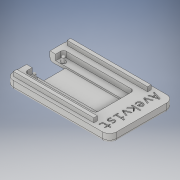
# Autodesk Inventor part: NodeMCU_Template
Saved by Autodesk Inventor 2019 (Build 230136000, 136)
## iProperties
Created: 2018-11-08
Part Number: NodeMCU_Template
Material: Generic
Document SubType Name: Modeling
Designer: hampu
Density: 1 g/cm^3
Appearance: Default
Author: hampu
Autodesk Inventor part; units mm, degrees
(part 1 of 2)
ref_plane "YZ Plane" through (0, 0, 0) normal (1, 0, 0) x (0, 1, 0)
ref_plane "XZ Plane" through (0, 0, 0) normal (0, 1, 0) x (-1, 0, 0)
ref_plane "XY Plane" through (0, 0, 0) normal (0, 0, 1) x (1, 0, 0)
sketch "Sketch1" plane through (0, 0, 0) normal (0, 1, 0) x (-1, 0, 0)
  line L0 (24.095, -12.775) -> (-24.095, -12.775)
  line L1 (-24.095, -12.775) -> (-24.095, 12.775)
  line L2 (-24.095, 12.775) -> (24.095, 12.775)
  line L3 (24.095, 12.775) -> (24.095, -12.775)
  line L4 (24.095, -12.775) -> (-24.095, 12.775) construction
  line L5 (-24.095, -12.775) -> (24.095, 12.775) construction
  line L6 (24.095, -12.775) -> (21.595, -12.775)
  line L7 (24.095, -12.775) -> (24.095, -10.275)
  line L8 (24.095, 12.775) -> (24.095, 10.275)
  line L9 (-24.095, -12.775) -> (-21.595, -12.775)
  line L10 (-24.095, 12.775) -> (-21.595, 12.775)
  line L11 (-24.095, 10.275) -> (-24.095, 12.775)
  circle A0 centre (21.595, -10.275) radius 1.7053
  circle A1 centre (-21.595, -10.275) radius 1.7053
  circle A2 centre (21.595, 10.275) radius 1.7053
  circle A3 centre (-21.595, 10.275) radius 1.7053
  point P0 (0, 0)
  dimension "d4" = 48.19
  dimension "d5" = 25.55
  dimension "d15" = 3.4106
  dimension "d18" = 43.19
  dimension "d21" = 20.55
  constraints: 24 end point, 4 centre point, 4 horizontal, 3 point on line, 2 midpoint, 2 parallel, 1 perpendicular, 1 vertical, 6 other
  measures "d4" distance of L0.start L0.end
  measures "d5" distance of L0.end L1.end
  measures "d15" diameter of A0
  measures "d18" distance of A0.centre A1.centre
  measures "d21" distance of A0.centre A2.centre
extrude "Extrusion2" add sketch "Sketch1" along normal blind 1.6
fillet "Fillet1" radius 2.5 4 edges at (-24.095, 0.8, 12.775) (-24.095, 0.8, -12.775) (24.095, 0.8, 12.775) (24.095, 0.8, -12.775)
sketch "Sketch3" plane through (0, 1.6, 0) normal (0, 1, 0) x (1, 0, 0)
  circle A0 centre (-21.595, 10.275) radius 1.7053 projected
  line L0 (21.595, 12.775) -> (-21.595, 12.775) projected
  line L1 (-19.1777, 12.775) -> (-18.624, 12.775) construction
  line L2 (-18.865, 12.2213) -> (-16.951, 12.2213)
  line L3 (-19.1777, 11.908) -> (-18.865, 12.2213)
  line L4 (-19.1777, 11.908) -> (-19.1777, 9.993)
  line L5 (-19.1777, 9.993) -> (-18.865, 9.6808)
  line L6 (-18.865, 9.6808) -> (-16.951, 9.6808)
  line L7 (-16.951, 9.6808) -> (-16.6393, 9.993)
  line L8 (-16.6393, 9.993) -> (-16.6393, 11.9102)
  line L9 (-18.226, 11.268) -> (-17.591, 11.268)
  line L10 (-17.591, 11.268) -> (-17.591, 10.633)
  line L11 (-17.591, 10.633) -> (-18.226, 10.633)
  line L12 (-18.226, 10.633) -> (-18.226, 11.268)
  line L13 (-16.951, 12.2213) -> (-16.6393, 11.9102)
  line L14 (-16.6377, 11.908) -> (-16.325, 12.2213)
  line L15 (-16.6377, 11.908) -> (-16.6377, 9.993)
  line L16 (-16.6377, 9.993) -> (-16.325, 9.6808)
  line L17 (-15.686, 10.633) -> (-15.686, 11.268)
  line L18 (-15.686, 11.268) -> (-15.051, 11.268)
  line L19 (-15.051, 11.268) -> (-15.051, 10.633)
  line L20 (-15.051, 10.633) -> (-15.686, 10.633)
  line L21 (-16.325, 9.6808) -> (-14.411, 9.6808)
  line L22 (-14.411, 9.6808) -> (-14.0993, 9.993)
  line L23 (-14.0993, 9.993) -> (-14.0993, 11.9102)
  line L24 (-14.411, 12.2213) -> (-14.0993, 11.9102)
  line L25 (-16.325, 12.2213) -> (-14.411, 12.2213)
  line L26 (-14.0977, 11.908) -> (-13.785, 12.2213)
  line L27 (-14.0977, 11.908) -> (-14.0977, 9.993)
  line L28 (-14.0977, 9.993) -> (-13.785, 9.6808)
  line L29 (-13.146, 10.633) -> (-13.146, 11.268)
  line L30 (-13.146, 11.268) -> (-12.511, 11.268)
  line L31 (-12.511, 11.268) -> (-12.511, 10.633)
  line L32 (-12.511, 10.633) -> (-13.146, 10.633)
  line L33 (-13.785, 9.6808) -> (-11.871, 9.6808)
  line L34 (-11.871, 9.6808) -> (-11.5593, 9.993)
  line L35 (-11.5593, 9.993) -> (-11.5593, 11.9102)
  line L36 (-11.871, 12.2213) -> (-11.5593, 11.9102)
  line L37 (-13.785, 12.2213) -> (-11.871, 12.2213)
  line L38 (-11.5577, 11.908) -> (-11.245, 12.2213)
  line L39 (-11.5577, 11.908) -> (-11.5577, 9.993)
  line L40 (-11.5577, 9.993) -> (-11.245, 9.6808)
  line L41 (-10.606, 10.633) -> (-10.606, 11.268)
  line L42 (-10.606, 11.268) -> (-9.971, 11.268)
  line L43 (-9.971, 11.268) -> (-9.971, 10.633)
  line L44 (-9.971, 10.633) -> (-10.606, 10.633)
  line L45 (-11.245, 9.6808) -> (-9.331, 9.6808)
  line L46 (-9.331, 9.6808) -> (-9.0193, 9.993)
  line L47 (-9.0193, 9.993) -> (-9.0193, 11.9102)
  line L48 (-9.331, 12.2213) -> (-9.0193, 11.9102)
  line L49 (-11.245, 12.2213) -> (-9.331, 12.2213)
  line L50 (-9.0177, 11.908) -> (-8.705, 12.2213)
  line L51 (-9.0177, 11.908) -> (-9.0177, 9.993)
  line L52 (-9.0177, 9.993) -> (-8.705, 9.6808)
  line L53 (-8.066, 10.633) -> (-8.066, 11.268)
  line L54 (-8.066, 11.268) -> (-7.431, 11.268)
  line L55 (-7.431, 11.268) -> (-7.431, 10.633)
  line L56 (-7.431, 10.633) -> (-8.066, 10.633)
  line L57 (-8.705, 9.6808) -> (-6.791, 9.6808)
  line L58 (-6.791, 9.6808) -> (-6.4793, 9.993)
  line L59 (-6.4793, 9.993) -> (-6.4793, 11.9102)
  line L60 (-6.791, 12.2213) -> (-6.4793, 11.9102)
  line L61 (-8.705, 12.2213) -> (-6.791, 12.2213)
  line L62 (-6.4777, 11.908) -> (-6.165, 12.2213)
  line L63 (-6.4777, 11.908) -> (-6.4777, 9.993)
  line L64 (-6.4777, 9.993) -> (-6.165, 9.6808)
  line L65 (-5.526, 10.633) -> (-5.526, 11.268)
  line L66 (-5.526, 11.268) -> (-4.891, 11.268)
  line L67 (-4.891, 11.268) -> (-4.891, 10.633)
  line L68 (-4.891, 10.633) -> (-5.526, 10.633)
  line L69 (-6.165, 9.6808) -> (-4.251, 9.6808)
  line L70 (-4.251, 9.6808) -> (-3.9393, 9.993)
  line L71 (-3.9393, 9.993) -> (-3.9393, 11.9102)
  line L72 (-4.251, 12.2213) -> (-3.9393, 11.9102)
  line L73 (-6.165, 12.2213) -> (-4.251, 12.2213)
  line L74 (-3.9377, 11.908) -> (-3.625, 12.2213)
  line L75 (-3.9377, 11.908) -> (-3.9377, 9.993)
  line L76 (-3.9377, 9.993) -> (-3.625, 9.6808)
  line L77 (-2.986, 10.633) -> (-2.986, 11.268)
  line L78 (-2.986, 11.268) -> (-2.351, 11.268)
  line L79 (-2.351, 11.268) -> (-2.351, 10.633)
  line L80 (-2.351, 10.633) -> (-2.986, 10.633)
  line L81 (-3.625, 9.6808) -> (-1.711, 9.6808)
  line L82 (-1.711, 9.6808) -> (-1.3993, 9.993)
  line L83 (-1.3993, 9.993) -> (-1.3993, 11.9102)
  line L84 (-1.711, 12.2213) -> (-1.3993, 11.9102)
  line L85 (-3.625, 12.2213) -> (-1.711, 12.2213)
  line L86 (-1.3977, 11.908) -> (-1.085, 12.2213)
  line L87 (-1.3977, 11.908) -> (-1.3977, 9.993)
  line L88 (-1.3977, 9.993) -> (-1.085, 9.6808)
  line L89 (-0.446, 10.633) -> (-0.446, 11.268)
  line L90 (-0.446, 11.268) -> (0.189, 11.268)
  line L91 (0.189, 11.268) -> (0.189, 10.633)
  line L92 (0.189, 10.633) -> (-0.446, 10.633)
  line L93 (-1.085, 9.6808) -> (0.829, 9.6808)
  line L94 (0.829, 9.6808) -> (1.1407, 9.993)
  line L95 (1.1407, 9.993) -> (1.1407, 11.9102)
  line L96 (0.829, 12.2213) -> (1.1407, 11.9102)
  line L97 (-1.085, 12.2213) -> (0.829, 12.2213)
  line L98 (1.1423, 11.908) -> (1.455, 12.2213)
  line L99 (1.1423, 11.908) -> (1.1423, 9.993)
  line L100 (1.1423, 9.993) -> (1.455, 9.6808)
  line L101 (2.094, 10.633) -> (2.094, 11.268)
  line L102 (2.094, 11.268) -> (2.729, 11.268)
  line L103 (2.729, 11.268) -> (2.729, 10.633)
  line L104 (2.729, 10.633) -> (2.094, 10.633)
  line L105 (1.455, 9.6808) -> (3.369, 9.6808)
  line L106 (3.369, 9.6808) -> (3.6807, 9.993)
  line L107 (3.6807, 9.993) -> (3.6807, 11.9102)
  line L108 (3.369, 12.2213) -> (3.6807, 11.9102)
  line L109 (1.455, 12.2213) -> (3.369, 12.2213)
  line L110 (3.6823, 11.908) -> (3.995, 12.2213)
  line L111 (3.6823, 11.908) -> (3.6823, 9.993)
  line L112 (3.6823, 9.993) -> (3.995, 9.6808)
  line L113 (4.634, 10.633) -> (4.634, 11.268)
  line L114 (4.634, 11.268) -> (5.269, 11.268)
  line L115 (5.269, 11.268) -> (5.269, 10.633)
  line L116 (5.269, 10.633) -> (4.634, 10.633)
  line L117 (3.995, 9.6808) -> (5.909, 9.6808)
  line L118 (5.909, 9.6808) -> (6.2207, 9.993)
  line L119 (6.2207, 9.993) -> (6.2207, 11.9102)
  line L120 (5.909, 12.2213) -> (6.2207, 11.9102)
  line L121 (3.995, 12.2213) -> (5.909, 12.2213)
  line L122 (6.2223, 11.908) -> (6.535, 12.2213)
  line L123 (6.2223, 11.908) -> (6.2223, 9.993)
  line L124 (6.2223, 9.993) -> (6.535, 9.6808)
  line L125 (7.174, 10.633) -> (7.174, 11.268)
  line L126 (7.174, 11.268) -> (7.809, 11.268)
  line L127 (7.809, 11.268) -> (7.809, 10.633)
  line L128 (7.809, 10.633) -> (7.174, 10.633)
  line L129 (6.535, 9.6808) -> (8.449, 9.6808)
  line L130 (8.449, 9.6808) -> (8.7607, 9.993)
  line L131 (8.7607, 9.993) -> (8.7607, 11.9102)
  line L132 (8.449, 12.2213) -> (8.7607, 11.9102)
  line L133 (6.535, 12.2213) -> (8.449, 12.2213)
  line L134 (8.7623, 11.908) -> (9.075, 12.2213)
  line L135 (8.7623, 11.908) -> (8.7623, 9.993)
  line L136 (8.7623, 9.993) -> (9.075, 9.6808)
  line L137 (9.714, 10.633) -> (9.714, 11.268)
  line L138 (9.714, 11.268) -> (10.349, 11.268)
  line L139 (10.349, 11.268) -> (10.349, 10.633)
  line L140 (10.349, 10.633) -> (9.714, 10.633)
  line L141 (9.075, 9.6808) -> (10.989, 9.6808)
  line L142 (10.989, 9.6808) -> (11.3007, 9.993)
  line L143 (11.3007, 9.993) -> (11.3007, 11.9102)
  line L144 (10.989, 12.2213) -> (11.3007, 11.9102)
  line L145 (9.075, 12.2213) -> (10.989, 12.2213)
  line L146 (11.3023, 11.908) -> (11.615, 12.2213)
  line L147 (11.3023, 11.908) -> (11.3023, 9.993)
  line L148 (11.3023, 9.993) -> (11.615, 9.6808)
  line L149 (12.254, 10.633) -> (12.254, 11.268)
  line L150 (12.254, 11.268) -> (12.889, 11.268)
  line L151 (12.889, 11.268) -> (12.889, 10.633)
  line L152 (12.889, 10.633) -> (12.254, 10.633)
  line L153 (11.615, 9.6808) -> (13.529, 9.6808)
  line L154 (13.529, 9.6808) -> (13.8407, 9.993)
  line L155 (13.8407, 9.993) -> (13.8407, 11.9102)
  line L156 (13.529, 12.2213) -> (13.8407, 11.9102)
  line L157 (11.615, 12.2213) -> (13.529, 12.2213)
  line L158 (13.8423, 11.908) -> (14.155, 12.2213)
  line L159 (13.8423, 11.908) -> (13.8423, 9.993)
  line L160 (13.8423, 9.993) -> (14.155, 9.6808)
  line L161 (14.794, 10.633) -> (14.794, 11.268)
  line L162 (14.794, 11.268) -> (15.429, 11.268)
  line L163 (15.429, 11.268) -> (15.429, 10.633)
  line L164 (15.429, 10.633) -> (14.794, 10.633)
  line L165 (14.155, 9.6808) -> (16.069, 9.6808)
  line L166 (16.069, 9.6808) -> (16.3807, 9.993)
  line L167 (16.3807, 9.993) -> (16.3807, 11.9102)
  line L168 (16.069, 12.2213) -> (16.3807, 11.9102)
  line L169 (14.155, 12.2213) -> (16.069, 12.2213)
  line L170 (16.3823, 11.908) -> (16.695, 12.2213)
  line L171 (16.3823, 11.908) -> (16.3823, 9.993)
  line L172 (16.3823, 9.993) -> (16.695, 9.6808)
  line L173 (17.334, 10.633) -> (17.334, 11.268)
  line L174 (17.334, 11.268) -> (17.969, 11.268)
  line L175 (17.969, 11.268) -> (17.969, 10.633)
  line L176 (17.969, 10.633) -> (17.334, 10.633)
  line L177 (16.695, 9.6808) -> (18.609, 9.6808)
  line L178 (18.609, 9.6808) -> (18.9207, 9.993)
  line L179 (18.9207, 9.993) -> (18.9207, 11.9102)
  line L180 (18.609, 12.2213) -> (18.9207, 11.9102)
  line L181 (16.695, 12.2213) -> (18.609, 12.2213)
  line L182 (-19.1777, -9.9934) -> (-18.865, -9.6801)
  line L183 (-19.1777, -9.9934) -> (-19.1777, -11.9084)
  line L184 (-19.1777, -11.9084) -> (-18.865, -12.2206)
  line L185 (-18.226, -11.2684) -> (-18.226, -10.6334)
  line L186 (-18.226, -10.6334) -> (-17.591, -10.6334)
  line L187 (-17.591, -10.6334) -> (-17.591, -11.2684)
  line L188 (-17.591, -11.2684) -> (-18.226, -11.2684)
  line L189 (-18.865, -12.2206) -> (-16.951, -12.2206)
  line L190 (-16.951, -12.2206) -> (-16.6393, -11.9084)
  line L191 (-16.6393, -11.9084) -> (-16.6393, -9.9912)
  line L192 (-16.951, -9.6801) -> (-16.6393, -9.9912)
  line L193 (-18.865, -9.6801) -> (-16.951, -9.6801)
  line L194 (-16.6377, -9.9934) -> (-16.325, -9.6801)
  line L195 (-16.6377, -9.9934) -> (-16.6377, -11.9084)
  line L196 (-16.6377, -11.9084) -> (-16.325, -12.2206)
  line L197 (-15.686, -11.2684) -> (-15.686, -10.6334)
  line L198 (-15.686, -10.6334) -> (-15.051, -10.6334)
  line L199 (-15.051, -10.6334) -> (-15.051, -11.2684)
  line L200 (-15.051, -11.2684) -> (-15.686, -11.2684)
  line L201 (-16.325, -12.2206) -> (-14.411, -12.2206)
  line L202 (-14.411, -12.2206) -> (-14.0993, -11.9084)
  line L203 (-14.0993, -11.9084) -> (-14.0993, -9.9912)
  line L204 (-14.411, -9.6801) -> (-14.0993, -9.9912)
  line L205 (-16.325, -9.6801) -> (-14.411, -9.6801)
  line L206 (-14.0977, -9.9934) -> (-13.785, -9.6801)
  line L207 (-14.0977, -9.9934) -> (-14.0977, -11.9084)
  line L208 (-14.0977, -11.9084) -> (-13.785, -12.2206)
  line L209 (-13.146, -11.2684) -> (-13.146, -10.6334)
  line L210 (-13.146, -10.6334) -> (-12.511, -10.6334)
  line L211 (-12.511, -10.6334) -> (-12.511, -11.2684)
  line L212 (-12.511, -11.2684) -> (-13.146, -11.2684)
  line L213 (-13.785, -12.2206) -> (-11.871, -12.2206)
  line L214 (-11.871, -12.2206) -> (-11.5593, -11.9084)
  line L215 (-11.5593, -11.9084) -> (-11.5593, -9.9912)
  line L216 (-11.871, -9.6801) -> (-11.5593, -9.9912)
  line L217 (-13.785, -9.6801) -> (-11.871, -9.6801)
  line L218 (-11.5577, -9.9934) -> (-11.245, -9.6801)
  line L219 (-11.5577, -9.9934) -> (-11.5577, -11.9084)
  line L220 (-11.5577, -11.9084) -> (-11.245, -12.2206)
  line L221 (-10.606, -11.2684) -> (-10.606, -10.6334)
  line L222 (-10.606, -10.6334) -> (-9.971, -10.6334)
  line L223 (-9.971, -10.6334) -> (-9.971, -11.2684)
  line L224 (-9.971, -11.2684) -> (-10.606, -11.2684)
  line L225 (-11.245, -12.2206) -> (-9.331, -12.2206)
  line L226 (-9.331, -12.2206) -> (-9.0193, -11.9084)
  line L227 (-9.0193, -11.9084) -> (-9.0193, -9.9912)
  line L228 (-9.331, -9.6801) -> (-9.0193, -9.9912)
  line L229 (-11.245, -9.6801) -> (-9.331, -9.6801)
  line L230 (-9.0177, -9.9934) -> (-8.705, -9.6801)
  line L231 (-9.0177, -9.9934) -> (-9.0177, -11.9084)
  line L232 (-9.0177, -11.9084) -> (-8.705, -12.2206)
  line L233 (-8.066, -11.2684) -> (-8.066, -10.6334)
  line L234 (-8.066, -10.6334) -> (-7.431, -10.6334)
  line L235 (-7.431, -10.6334) -> (-7.431, -11.2684)
  line L236 (-7.431, -11.2684) -> (-8.066, -11.2684)
  line L237 (-8.705, -12.2206) -> (-6.791, -12.2206)
  line L238 (-6.791, -12.2206) -> (-6.4793, -11.9084)
  line L239 (-6.4793, -11.9084) -> (-6.4793, -9.9912)
  line L240 (-6.791, -9.6801) -> (-6.4793, -9.9912)
  line L241 (-8.705, -9.6801) -> (-6.791, -9.6801)
  line L242 (-6.4777, -9.9934) -> (-6.165, -9.6801)
  line L243 (-6.4777, -9.9934) -> (-6.4777, -11.9084)
  line L244 (-6.4777, -11.9084) -> (-6.165, -12.2206)
  line L245 (-5.526, -11.2684) -> (-5.526, -10.6334)
  line L246 (-5.526, -10.6334) -> (-4.891, -10.6334)
  line L247 (-4.891, -10.6334) -> (-4.891, -11.2684)
  line L248 (-4.891, -11.2684) -> (-5.526, -11.2684)
  line L249 (-6.165, -12.2206) -> (-4.251, -12.2206)
  line L250 (-4.251, -12.2206) -> (-3.9393, -11.9084)
  line L251 (-3.9393, -11.9084) -> (-3.9393, -9.9912)
  line L252 (-4.251, -9.6801) -> (-3.9393, -9.9912)
  line L253 (-6.165, -9.6801) -> (-4.251, -9.6801)
  line L254 (-3.9377, -9.9934) -> (-3.625, -9.6801)
  line L255 (-3.9377, -9.9934) -> (-3.9377, -11.9084)
  line L256 (-3.9377, -11.9084) -> (-3.625, -12.2206)
  line L257 (-2.986, -11.2684) -> (-2.986, -10.6334)
  line L258 (-2.986, -10.6334) -> (-2.351, -10.6334)
  line L259 (-2.351, -10.6334) -> (-2.351, -11.2684)
  line L260 (-2.351, -11.2684) -> (-2.986, -11.2684)
  line L261 (-3.625, -12.2206) -> (-1.711, -12.2206)
  line L262 (-1.711, -12.2206) -> (-1.3993, -11.9084)
  line L263 (-1.3993, -11.9084) -> (-1.3993, -9.9912)
  line L264 (-1.711, -9.6801) -> (-1.3993, -9.9912)
  line L265 (-3.625, -9.6801) -> (-1.711, -9.6801)
  line L266 (-1.3977, -9.9934) -> (-1.085, -9.6801)
  line L267 (-1.3977, -9.9934) -> (-1.3977, -11.9084)
  line L268 (-1.3977, -11.9084) -> (-1.085, -12.2206)
  line L269 (-0.446, -11.2684) -> (-0.446, -10.6334)
  line L270 (-0.446, -10.6334) -> (0.189, -10.6334)
  line L271 (0.189, -10.6334) -> (0.189, -11.2684)
  line L272 (0.189, -11.2684) -> (-0.446, -11.2684)
  line L273 (-1.085, -12.2206) -> (0.829, -12.2206)
  line L274 (0.829, -12.2206) -> (1.1407, -11.9084)
  line L275 (1.1407, -11.9084) -> (1.1407, -9.9912)
  line L276 (0.829, -9.6801) -> (1.1407, -9.9912)
  line L277 (-1.085, -9.6801) -> (0.829, -9.6801)
  line L278 (1.1423, -9.9934) -> (1.455, -9.6801)
  line L279 (1.1423, -9.9934) -> (1.1423, -11.9084)
  line L280 (1.1423, -11.9084) -> (1.455, -12.2206)
  line L281 (2.094, -11.2684) -> (2.094, -10.6334)
  line L282 (2.094, -10.6334) -> (2.729, -10.6334)
  line L283 (2.729, -10.6334) -> (2.729, -11.2684)
  line L284 (2.729, -11.2684) -> (2.094, -11.2684)
  line L285 (1.455, -12.2206) -> (3.369, -12.2206)
  line L286 (3.369, -12.2206) -> (3.6807, -11.9084)
  line L287 (3.6807, -11.9084) -> (3.6807, -9.9912)
  line L288 (3.369, -9.6801) -> (3.6807, -9.9912)
  line L289 (1.455, -9.6801) -> (3.369, -9.6801)
  line L290 (3.6823, -9.9934) -> (3.995, -9.6801)
  line L291 (3.6823, -9.9934) -> (3.6823, -11.9084)
  line L292 (3.6823, -11.9084) -> (3.995, -12.2206)
  line L293 (4.634, -11.2684) -> (4.634, -10.6334)
  line L294 (4.634, -10.6334) -> (5.269, -10.6334)
  line L295 (5.269, -10.6334) -> (5.269, -11.2684)
  line L296 (5.269, -11.2684) -> (4.634, -11.2684)
  line L297 (3.995, -12.2206) -> (5.909, -12.2206)
  line L298 (5.909, -12.2206) -> (6.2207, -11.9084)
  line L299 (6.2207, -11.9084) -> (6.2207, -9.9912)
  line L300 (5.909, -9.6801) -> (6.2207, -9.9912)
  line L301 (3.995, -9.6801) -> (5.909, -9.6801)
  line L302 (6.2223, -9.9934) -> (6.535, -9.6801)
  line L303 (6.2223, -9.9934) -> (6.2223, -11.9084)
  line L304 (6.2223, -11.9084) -> (6.535, -12.2206)
  line L305 (7.174, -11.2684) -> (7.174, -10.6334)
  line L306 (7.174, -10.6334) -> (7.809, -10.6334)
  line L307 (7.809, -10.6334) -> (7.809, -11.2684)
  line L308 (7.809, -11.2684) -> (7.174, -11.2684)
  line L309 (6.535, -12.2206) -> (8.449, -12.2206)
  line L310 (8.449, -12.2206) -> (8.7607, -11.9084)
  line L311 (8.7607, -11.9084) -> (8.7607, -9.9912)
  line L312 (8.449, -9.6801) -> (8.7607, -9.9912)
  line L313 (6.535, -9.6801) -> (8.449, -9.6801)
  line L314 (8.7623, -9.9934) -> (9.075, -9.6801)
  line L315 (8.7623, -9.9934) -> (8.7623, -11.9084)
  line L316 (8.7623, -11.9084) -> (9.075, -12.2206)
  line L317 (9.714, -11.2684) -> (9.714, -10.6334)
  line L318 (9.714, -10.6334) -> (10.349, -10.6334)
  line L319 (10.349, -10.6334) -> (10.349, -11.2684)
  line L320 (10.349, -11.2684) -> (9.714, -11.2684)
  line L321 (9.075, -12.2206) -> (10.989, -12.2206)
  line L322 (10.989, -12.2206) -> (11.3007, -11.9084)
  line L323 (11.3007, -11.9084) -> (11.3007, -9.9912)
  line L324 (10.989, -9.6801) -> (11.3007, -9.9912)
  line L325 (9.075, -9.6801) -> (10.989, -9.6801)
  line L326 (11.3023, -9.9934) -> (11.615, -9.6801)
  line L327 (11.3023, -9.9934) -> (11.3023, -11.9084)
  line L328 (11.3023, -11.9084) -> (11.615, -12.2206)
  line L329 (12.254, -11.2684) -> (12.254, -10.6334)
  line L330 (12.254, -10.6334) -> (12.889, -10.6334)
  line L331 (12.889, -10.6334) -> (12.889, -11.2684)
  line L332 (12.889, -11.2684) -> (12.254, -11.2684)
  line L333 (11.615, -12.2206) -> (13.529, -12.2206)
  line L334 (13.529, -12.2206) -> (13.8407, -11.9084)
  line L335 (13.8407, -11.9084) -> (13.8407, -9.9912)
  line L336 (13.529, -9.6801) -> (13.8407, -9.9912)
  line L337 (11.615, -9.6801) -> (13.529, -9.6801)
  line L338 (13.8423, -9.9934) -> (14.155, -9.6801)
  line L339 (13.8423, -9.9934) -> (13.8423, -11.9084)
  line L340 (13.8423, -11.9084) -> (14.155, -12.2206)
  line L341 (14.794, -11.2684) -> (14.794, -10.6334)
  line L342 (14.794, -10.6334) -> (15.429, -10.6334)
  line L343 (15.429, -10.6334) -> (15.429, -11.2684)
  line L344 (15.429, -11.2684) -> (14.794, -11.2684)
  line L345 (14.155, -12.2206) -> (16.069, -12.2206)
  line L346 (16.069, -12.2206) -> (16.3807, -11.9084)
  line L347 (16.3807, -11.9084) -> (16.3807, -9.9912)
  line L348 (16.069, -9.6801) -> (16.3807, -9.9912)
  line L349 (14.155, -9.6801) -> (16.069, -9.6801)
  line L350 (16.3823, -9.9934) -> (16.695, -9.6801)
  line L351 (16.3823, -9.9934) -> (16.3823, -11.9084)
  line L352 (16.3823, -11.9084) -> (16.695, -12.2206)
  line L353 (17.334, -11.2684) -> (17.334, -10.6334)
  line L354 (17.334, -10.6334) -> (17.969, -10.6334)
  line L355 (17.969, -10.6334) -> (17.969, -11.2684)
  line L356 (17.969, -11.2684) -> (17.334, -11.2684)
  line L357 (16.695, -12.2206) -> (18.609, -12.2206)
  line L358 (18.609, -12.2206) -> (18.9207, -11.9084)
  line L359 (18.9207, -11.9084) -> (18.9207, -9.9912)
  line L360 (18.609, -9.6801) -> (18.9207, -9.9912)
  line L361 (16.695, -9.6801) -> (18.609, -9.6801)
  point P0 (0, 0)
  dimension "d71" = 1.914
  dimension "d72" = 1.915
  dimension "d73" = 0.635
  dimension "d74" = 0.635
  dimension "d77" = 2.54
  dimension "d80" = 21.9014
  constraints: 722 end point, 4 horizontal, 4 perpendicular, 3 parallel, 2 collinear, 2 vertical, 1 point on line, 694 other
  measures "d71" distance of L2.start L2.end
  measures "d72" distance of L3.start L4.end
  measures "d73" distance of L10.end L11.end
  measures "d74" distance of L9.end L10.end
  measures "d77" distance of L3.start L14.start
  measures "d80" distance of L3.start L182.start
extrude "Extrusion3" add sketch "Sketch3" along normal blind 1.905 contours L2 L13 L8 L7 L6 L5 L4 L3 | L14 L25 L24 L23 L22 L21 L16 L8 | L26 L37 L36 L35 L34 L33 L28 L23 | L38 L49 L48 L47 L46 L45 L40 L35 | L50 L61 L60 L59 L58 L57 L52 L47 | L62 L73 L72 L71 L70 L69 L64 L59 | L74 L85 L84 L83 L82 L81 L76 L71 | L86 L97 L96 L95 L94 L93 L88 L83 | L98 L109 L108 L107 L106 L105 L100 L95 | L110 L121 L120 L119 L118 L117 L112 L107 | L122 L133 L132 L131 L130 L129 L124 L119 | L134 L145 L144 L143 L142 L141 L136 L131 | L146 L157 L156 L155 L154 L153 L148 L143 | L158 L169 L168 L167 L166 L165 L160 L155 | L170 L181 L180 L179 L178 L177 L172 L167 | L182 L193 L192 L191 L190 L189 L184 L183 | L194 L205 L204 L203 L202 L201 L196 L191 | L206 L217 L216 L215 L214 L213 L208 L203 | L218 L229 L228 L227 L226 L225 L220 L215 | L230 L241 L240 L239 L238 L237 L232 L227 | L242 L253 L252 L251 L250 L249 L244 L239 | L254 L265 L264 L263 L262 L261 L256 L251 | L266 L277 L276 L275 L274 L273 L268 L263 | L278 L289 L288 L287 L286 L285 L280 L275 | L290 L301 L300 L299 L298 L297 L292 L287 | L302 L313 L312 L311 L310 L309 L304 L299 | L314 L325 L324 L323 L322 L321 L316 L311 | L326 L337 L336 L335 L334 L333 L328 L323 | L338 L349 L348 L347 L346 L345 L340 L335 | L350 L361 L360 L359 L358 L357 L352 L347
sketch "Sketch4" plane through (0, 3.505, 0) normal (0, 1, 0) x (1, 0, 0)
  line L0 (-18.226, 10.633) -> (-18.226, 11.268) projected
  line L1 (-17.591, 10.633) -> (-17.591, 11.268) projected
  line L2 (-18.226, 11.268) -> (-17.591, 11.268)
  line L3 (-17.591, 11.268) -> (-17.591, 10.633)
  line L4 (-17.591, 10.633) -> (-18.226, 10.633)
  line L5 (-18.226, 10.633) -> (-18.226, 11.268)
  line L6 (-15.051, 11.268) -> (-15.051, 10.633)
  line L7 (-15.686, 11.268) -> (-15.051, 11.268)
  line L8 (-15.686, 10.633) -> (-15.686, 11.268)
  line L9 (-15.051, 10.633) -> (-15.686, 10.633)
  line L10 (-12.511, 11.268) -> (-12.511, 10.633)
  line L11 (-13.146, 11.268) -> (-12.511, 11.268)
  line L12 (-13.146, 10.633) -> (-13.146, 11.268)
  line L13 (-12.511, 10.633) -> (-13.146, 10.633)
  line L14 (-9.971, 11.268) -> (-9.971, 10.633)
  line L15 (-10.606, 11.268) -> (-9.971, 11.268)
  line L16 (-10.606, 10.633) -> (-10.606, 11.268)
  line L17 (-9.971, 10.633) -> (-10.606, 10.633)
  line L18 (-7.431, 11.268) -> (-7.431, 10.633)
  line L19 (-8.066, 11.268) -> (-7.431, 11.268)
  line L20 (-8.066, 10.633) -> (-8.066, 11.268)
  line L21 (-7.431, 10.633) -> (-8.066, 10.633)
  line L22 (-4.891, 11.268) -> (-4.891, 10.633)
  line L23 (-5.526, 11.268) -> (-4.891, 11.268)
  line L24 (-5.526, 10.633) -> (-5.526, 11.268)
  line L25 (-4.891, 10.633) -> (-5.526, 10.633)
  line L26 (-2.351, 11.268) -> (-2.351, 10.633)
  line L27 (-2.986, 11.268) -> (-2.351, 11.268)
  line L28 (-2.986, 10.633) -> (-2.986, 11.268)
  line L29 (-2.351, 10.633) -> (-2.986, 10.633)
  line L30 (0.189, 11.268) -> (0.189, 10.633)
  line L31 (-0.446, 11.268) -> (0.189, 11.268)
  line L32 (-0.446, 10.633) -> (-0.446, 11.268)
  line L33 (0.189, 10.633) -> (-0.446, 10.633)
  line L34 (2.729, 11.268) -> (2.729, 10.633)
  line L35 (2.094, 11.268) -> (2.729, 11.268)
  line L36 (2.094, 10.633) -> (2.094, 11.268)
  line L37 (2.729, 10.633) -> (2.094, 10.633)
  line L38 (5.269, 11.268) -> (5.269, 10.633)
  line L39 (4.634, 11.268) -> (5.269, 11.268)
  line L40 (4.634, 10.633) -> (4.634, 11.268)
  line L41 (5.269, 10.633) -> (4.634, 10.633)
  line L42 (7.809, 11.268) -> (7.809, 10.633)
  line L43 (7.174, 11.268) -> (7.809, 11.268)
  line L44 (7.174, 10.633) -> (7.174, 11.268)
  line L45 (7.809, 10.633) -> (7.174, 10.633)
  line L46 (10.349, 11.268) -> (10.349, 10.633)
  line L47 (9.714, 11.268) -> (10.349, 11.268)
  line L48 (9.714, 10.633) -> (9.714, 11.268)
  line L49 (10.349, 10.633) -> (9.714, 10.633)
  line L50 (12.889, 11.268) -> (12.889, 10.633)
  line L51 (12.254, 11.268) -> (12.889, 11.268)
  line L52 (12.254, 10.633) -> (12.254, 11.268)
  line L53 (12.889, 10.633) -> (12.254, 10.633)
  line L54 (15.429, 11.268) -> (15.429, 10.633)
  line L55 (14.794, 11.268) -> (15.429, 11.268)
  line L56 (14.794, 10.633) -> (14.794, 11.268)
  line L57 (15.429, 10.633) -> (14.794, 10.633)
  line L58 (17.969, 11.268) -> (17.969, 10.633)
  line L59 (17.334, 11.268) -> (17.969, 11.268)
  line L60 (17.334, 10.633) -> (17.334, 11.268)
  line L61 (17.969, 10.633) -> (17.334, 10.633)
  line L62 (-17.591, -10.6334) -> (-17.591, -11.2684)
  line L63 (-18.226, -10.6334) -> (-17.591, -10.6334)
  line L64 (-18.226, -11.2684) -> (-18.226, -10.6334)
  line L65 (-17.591, -11.2684) -> (-18.226, -11.2684)
  line L66 (-15.051, -10.6334) -> (-15.051, -11.2684)
  line L67 (-15.686, -10.6334) -> (-15.051, -10.6334)
  line L68 (-15.686, -11.2684) -> (-15.686, -10.6334)
  line L69 (-15.051, -11.2684) -> (-15.686, -11.2684)
  line L70 (-12.511, -10.6334) -> (-12.511, -11.2684)
  line L71 (-13.146, -10.6334) -> (-12.511, -10.6334)
  line L72 (-13.146, -11.2684) -> (-13.146, -10.6334)
  line L73 (-12.511, -11.2684) -> (-13.146, -11.2684)
  line L74 (-9.971, -10.6334) -> (-9.971, -11.2684)
  line L75 (-10.606, -10.6334) -> (-9.971, -10.6334)
  line L76 (-10.606, -11.2684) -> (-10.606, -10.6334)
  line L77 (-9.971, -11.2684) -> (-10.606, -11.2684)
  line L78 (-7.431, -10.6334) -> (-7.431, -11.2684)
  line L79 (-8.066, -10.6334) -> (-7.431, -10.6334)
  line L80 (-8.066, -11.2684) -> (-8.066, -10.6334)
  line L81 (-7.431, -11.2684) -> (-8.066, -11.2684)
  line L82 (-4.891, -10.6334) -> (-4.891, -11.2684)
  line L83 (-5.526, -10.6334) -> (-4.891, -10.6334)
  line L84 (-5.526, -11.2684) -> (-5.526, -10.6334)
  line L85 (-4.891, -11.2684) -> (-5.526, -11.2684)
  line L86 (-2.351, -10.6334) -> (-2.351, -11.2684)
  line L87 (-2.986, -10.6334) -> (-2.351, -10.6334)
  line L88 (-2.986, -11.2684) -> (-2.986, -10.6334)
  line L89 (-2.351, -11.2684) -> (-2.986, -11.2684)
  line L90 (0.189, -10.6334) -> (0.189, -11.2684)
  line L91 (-0.446, -10.6334) -> (0.189, -10.6334)
  line L92 (-0.446, -11.2684) -> (-0.446, -10.6334)
  line L93 (0.189, -11.2684) -> (-0.446, -11.2684)
  line L94 (2.729, -10.6334) -> (2.729, -11.2684)
  line L95 (2.094, -10.6334) -> (2.729, -10.6334)
  line L96 (2.094, -11.2684) -> (2.094, -10.6334)
  line L97 (2.729, -11.2684) -> (2.094, -11.2684)
  line L98 (5.269, -10.6334) -> (5.269, -11.2684)
  line L99 (4.634, -10.6334) -> (5.269, -10.6334)
  line L100 (4.634, -11.2684) -> (4.634, -10.6334)
  line L101 (5.269, -11.2684) -> (4.634, -11.2684)
  line L102 (7.809, -10.6334) -> (7.809, -11.2684)
  line L103 (7.174, -10.6334) -> (7.809, -10.6334)
  line L104 (7.174, -11.2684) -> (7.174, -10.6334)
  line L105 (7.809, -11.2684) -> (7.174, -11.2684)
  line L106 (10.349, -10.6334) -> (10.349, -11.2684)
  line L107 (9.714, -10.6334) -> (10.349, -10.6334)
  line L108 (9.714, -11.2684) -> (9.714, -10.6334)
  line L109 (10.349, -11.2684) -> (9.714, -11.2684)
  line L110 (12.889, -10.6334) -> (12.889, -11.2684)
  line L111 (12.254, -10.6334) -> (12.889, -10.6334)
  line L112 (12.254, -11.2684) -> (12.254, -10.6334)
  line L113 (12.889, -11.2684) -> (12.254, -11.2684)
  line L114 (15.429, -10.6334) -> (15.429, -11.2684)
  line L115 (14.794, -10.6334) -> (15.429, -10.6334)
  line L116 (14.794, -11.2684) -> (14.794, -10.6334)
  line L117 (15.429, -11.2684) -> (14.794, -11.2684)
  line L118 (17.969, -10.6334) -> (17.969, -11.2684)
  line L119 (17.334, -10.6334) -> (17.969, -10.6334)
  line L120 (17.334, -11.2684) -> (17.334, -10.6334)
  line L121 (17.969, -11.2684) -> (17.334, -11.2684)
  point P0 (0, 0)
  dimension "d89" = 2.54
  dimension "d92" = 21.9014
  constraints: 240 end point, 2 horizontal, 2 parallel, 1 collinear, 1 perpendicular, 1 vertical, 231 other
  measures "d89" distance of L2.end L6.start
  measures "d92" distance of L2.end L62.start
extrude "Extrusion5" add sketch "Sketch4" along normal blind 6.1913
chamfer "Chamfer1" distance 0.2 angle 45 120 edges at (-17.591, 9.6963, 10.9509) (-18.226, 9.6963, 10.9509) (-17.9085, 9.6963, 11.2684) (-17.9085, 9.6963, 10.6334) (-15.686, 9.6963, 10.9509) (-15.3685, 9.6963, 11.2684) (-15.051, 9.6963, 10.9509) (-15.3685, 9.6963, 10.6334) (-13.146, 9.6963, 10.9509) (-12.8285, 9.6963, 10.6334) (-12.511, 9.6963, 10.9509) (-12.8285, 9.6963, 11.2684) (-10.606, 9.6963, 10.9509) (-10.2885, 9.6963, 11.2684) (-9.971, 9.6963, 10.9509) (-10.2885, 9.6963, 10.6334) (-7.431, 9.6963, 10.9509) (-7.7485, 9.6963, 11.2684) (-8.066, 9.6963, 10.9509) (-7.7485, 9.6963, 10.6334) (-5.526, 9.6963, 10.9509) (-5.2085, 9.6963, 10.6334) (-4.891, 9.6963, 10.9509) (-5.2085, 9.6963, 11.2684) (-2.986, 9.6963, 10.9509) (-2.6685, 9.6963, 10.6334) (-2.6685, 9.6963, 11.2684) (-2.351, 9.6963, 10.9509) (-0.446, 9.6963, 10.9509) (-0.1285, 9.6963, 10.6334) (0.189, 9.6963, 10.9509) (-0.1285, 9.6963, 11.2684) (2.4115, 9.6963, 11.2684) (2.094, 9.6963, 10.9509) (2.4115, 9.6963, 10.6334) (2.729, 9.6963, 10.9509) (5.269, 9.6963, 10.9509) (4.9515, 9.6963, 11.2684) (4.634, 9.6963, 10.9509) (4.9515, 9.6963, 10.6334) (7.809, 9.6963, 10.9509) (7.4915, 9.6963, 11.2684) (7.174, 9.6963, 10.9509) (7.4915, 9.6963, 10.6334) (9.714, 9.6963, 10.9509) (10.0315, 9.6963, 10.6334) (10.349, 9.6963, 10.9509) (10.0315, 9.6963, 11.2684) (12.5715, 9.6963, 11.2684) (12.889, 9.6963, 10.9509) (12.5715, 9.6963, 10.6334) (12.254, 9.6963, 10.9509) (14.794, 9.6963, 10.9509) (15.1115, 9.6963, 10.6334) (15.429, 9.6963, 10.9509) (15.1115, 9.6963, 11.2684) (17.6515, 9.6963, 11.2684) (17.969, 9.6963, 10.9509) (17.6515, 9.6963, 10.6334) (17.334, 9.6963, 10.9509) (-18.226, 9.6963, -10.9505) (-17.9085, 9.6963, -11.268) (-17.591, 9.6963, -10.9505) (-17.9085, 9.6963, -10.633) (-15.686, 9.6963, -10.9505) (-15.3685, 9.6963, -11.268) (-15.051, 9.6963, -10.9505) (-15.3685, 9.6963, -10.633) (-13.146, 9.6963, -10.9505) (-12.8285, 9.6963, -11.268) (-12.511, 9.6963, -10.9505) (-12.8285, 9.6963, -10.633) (-10.606, 9.6963, -10.9505) (-10.2885, 9.6963, -10.633) (-9.971, 9.6963, -10.9505) (-10.2885, 9.6963, -11.268) (-8.066, 9.6963, -10.9505) (-7.7485, 9.6963, -11.268) (-7.431, 9.6963, -10.9505) (-7.7485, 9.6963, -10.633) (-5.526, 9.6963, -10.9505) (-5.2085, 9.6963, -10.633) (-4.891, 9.6963, -10.9505) (-5.2085, 9.6963, -11.268) (-2.986, 9.6963, -10.9505) (-2.6685, 9.6963, -10.633) (-2.6685, 9.6963, -11.268) (-2.351, 9.6963, -10.9505) (-0.446, 9.6963, -10.9505) (-0.1285, 9.6963, -11.268) (0.189, 9.6963, -10.9505) (-0.1285, 9.6963, -10.633) (2.094, 9.6963, -10.9505) (2.4115, 9.6963, -11.268) (2.729, 9.6963, -10.9505) (2.4115, 9.6963, -10.633) (4.634, 9.6963, -10.9505) (4.9515, 9.6963, -11.268) (4.9515, 9.6963, -10.633) (5.269, 9.6963, -10.9505) (7.174, 9.6963, -10.9505) (7.4915, 9.6963, -10.633) (7.809, 9.6963, -10.9505) (7.4915, 9.6963, -11.268) (10.0315, 9.6963, -11.268) (9.714, 9.6963, -10.9505) (10.0315, 9.6963, -10.633) (10.349, 9.6963, -10.9505) (12.254, 9.6963, -10.9505) (12.5715, 9.6963, -11.268) (12.5715, 9.6963, -10.633) (12.889, 9.6963, -10.9505) (15.1115, 9.6963, -11.268) (15.429, 9.6963, -10.9505) (15.1115, 9.6963, -10.633) (14.794, 9.6963, -10.9505) (17.334, 9.6963, -10.9505) (17.6515, 9.6963, -10.633) (17.969, 9.6963, -10.9505) (17.6515, 9.6963, -11.268)
sketch "Sketch5" plane through (0, 0, 0) normal (0, -1, 0) x (1, 0, 0)
  line L0 (17.5, -10) -> (-17.5, -10)
  line L1 (-17.5, -10) -> (-17.5, 10)
  line L2 (-17.5, 10) -> (17.5, 10)
  line L3 (17.5, 10) -> (17.5, -10)
  line L4 (17.5, -10) -> (-17.5, 10) construction
  line L5 (-17.5, -10) -> (17.5, 10) construction
  point P0 (0, 0)
  dimension "d100" = 35
  dimension "d101" = 20
  constraints: 12 end point, 2 midpoint, 2 parallel, 1 horizontal, 1 perpendicular
  measures "d100" distance of L1.end L2.end
  measures "d101" distance of L0.end L1.end
extrude "Extrusion6" add sketch "Sketch5" along normal blind 2.5
sketch "Sketch6" plane through (0, -2.5, 0) normal (0, -1, 0) x (1, 0, 0)
  line L0 (24.095, -12.775) -> (-24.095, -12.775)
  line L1 (-24.095, -12.775) -> (-24.095, 12.775)
  line L2 (-24.095, 12.775) -> (24.095, 12.775)
  line L3 (24.095, 12.775) -> (24.095, -12.775)
  line L4 (24.095, -12.775) -> (-24.095, 12.775) construction
  line L5 (-24.095, -12.775) -> (24.095, 12.775) construction
  point P0 (0, 0)
  constraints: 12 end point, 2 midpoint, 2 parallel, 1 horizontal, 1 perpendicular
extrude "Extrusion7" add sketch "Sketch6" against normal blind 3
sketch "Sketch7" plane through (-21.595, 0.5, -10.275) normal (0, 1, 0) x (1, 0, 0)
  circle A0 centre (0, 0) radius 1.7053
  circle A1 centre (0, -20.55) radius 1.7053 projected
  circle A2 centre (0, -20.55) radius 1.7053
  point P0 (21.595, -10.275)
  constraints: 2 centre point, 1 coincident
extrude "Extrusion8" cut sketch "Sketch7" against normal blind 3
sketch "Sketch8" plane through (-24.095, 1.6, -10.275) normal (-1, 0, 0) x (0, 0, 1)
  line L0 (-2.5, -4.1) -> (23.05, -4.1) projected
  line L1 (2, -2) -> (18.55, -2)
  line L2 (18.55, -2) -> (18.55, -4.1)
  line L3 (18.55, -4.1) -> (2, -4.1)
  line L4 (2, -4.1) -> (2, -2)
  point P0 (10.275, -1.6)
  dimension "d108" = 16.55
  constraints: 8 end point, 2 parallel, 1 horizontal, 1 perpendicular, 1 point on line
  measures "d108" distance of L2.end L3.end
extrude "Extrusion9" cut sketch "Sketch8" against normal blind 8
sketch "Sketch9" plane through (-24.095, 1.6, -10.275) normal (-1, 0, 0) x (0, 0, 1)
  line L0 (-2.5, -4.1) -> (2, -4.1) projected
  line L1 (23.05, -1.1) -> (23.05, 0) projected
  line L2 (-2.5, -4.1) -> (23.05, -4.1)
  line L3 (23.05, -4.1) -> (23.05, 0)
  line L4 (23.05, 0) -> (-2.5, 0)
  line L5 (-2.5, 0) -> (-2.5, -4.1)
  point P0 (10.275, -1.6)
  constraints: 8 end point, 2 parallel, 1 horizontal, 1 perpendicular
extrude "Extrusion10" add sketch "Sketch9" along normal blind 5
sketch "Sketch10" plane through (-24.095, 1.6, -10.275) normal (1, 0, 0) x (0, 0, -1)
  line L0 (-2, -4.1) -> (-2, -2) projected
  line L1 (-2, -4.1) -> (-18.55, -4.1)
  line L2 (-18.55, -4.1) -> (-18.55, -2)
  line L3 (-18.55, -2) -> (-2, -2)
  line L4 (-2, -2) -> (-2, -4.1)
  point P0 (-10.275, -1.6)
  constraints: 8 end point, 2 parallel, 1 horizontal, 1 perpendicular
extrude "Extrusion11" cut sketch "Sketch10" against normal blind 5
sketch "Sketch11" plane through (24.095, 1.6, 10.275) normal (1, 0, 0) x (0, 0, -1)
  line L0 (-2.5, -4.1) -> (23.05, -4.1) projected
  line L1 (-2.5, -4.1) -> (-2.5, 0) projected
  line L2 (23.05, -4.1) -> (-2.5, -4.1)
  line L3 (-2.5, -4.1) -> (-2.5, 0)
  line L4 (-2.5, 0) -> (23.05, 0)
  line L5 (23.05, 0) -> (23.05, -4.1)
  point P0 (10.275, -1.6)
  constraints: 8 end point, 2 parallel, 1 horizontal, 1 perpendicular
extrude "Extrusion12" add sketch "Sketch11" along normal blind 5
sketch "Sketch12" plane through (-21.595, 1.6, 12.775) normal (0, 0, 1) x (1, 0, 0)
  line L0 (-7.5, 0) -> (50.69, 0)
  line L1 (50.69, 0) -> (50.69, -4.1)
  line L2 (50.69, -4.1) -> (-7.5, -4.1)
  line L3 (-7.5, -4.1) -> (-7.5, 0)
  point P0 (21.595, -1.6)
  constraints: 8 end point, 2 parallel, 1 horizontal, 1 perpendicular
extrude "Extrusion13" add sketch "Sketch12" along normal blind 5
sketch "Sketch13" plane through (21.595, 1.6, -12.775) normal (0, 0, -1) x (-1, 0, 0)
  line L0 (-7.5, 0) -> (50.69, 0) projected
  line L1 (50.69, -4.1) -> (-7.5, -4.1) projected
  line L2 (-7.5, 0) -> (50.69, 0)
  line L3 (50.69, 0) -> (50.69, -4.1)
  line L4 (50.69, -4.1) -> (-7.5, -4.1)
  line L5 (-7.5, -4.1) -> (-7.5, 0)
  point P0 (21.595, -1.6)
  constraints: 8 end point, 2 parallel, 1 horizontal, 1 perpendicular
extrude "Extrusion14" add sketch "Sketch13" along normal blind 5
sketch "Sketch14" plane through (0, 1.6, 0) normal (0, 1, 0) x (1, 0, 0)
  line L0 (24.095, 10.275) -> (24.095, 12.775) projected
  line L1 (-24.095, -12.775) -> (24.095, -12.775)
  line L2 (24.095, -12.775) -> (24.095, 12.775)
  line L3 (24.095, 12.775) -> (-24.095, 12.775)
  line L4 (-24.095, 12.775) -> (-24.095, -12.775)
  line L5 (-24.095, -12.775) -> (24.095, 12.775) construction
  line L6 (24.095, -12.775) -> (-24.095, 12.775) construction
  point P0 (0, 0)
  constraints: 12 end point, 2 midpoint, 2 parallel, 1 horizontal, 1 perpendicular
extrude "Extrusion15" cut sketch "Sketch14" along normal blind 10
sketch "Sketch15" plane through (0, 1.6, 0) normal (0, 1, 0) x (1, 0, 0)
  line L0 (24.095, 12.775) -> (24.095, 10.275) projected
  line L1 (-24.095, -12.775) -> (24.095, 12.775) construction
  line L2 (24.095, -12.775) -> (-24.095, 12.775) construction
  line L3 (25.095, -13.775) -> (-25.095, -13.775)
  line L4 (-25.095, -13.775) -> (-25.095, 13.775)
  line L5 (-25.095, 13.775) -> (25.095, 13.775)
  line L6 (25.095, 13.775) -> (25.095, -13.775)
  point P0 (0, 0)
  constraints: 12 end point, 2 midpoint, 2 parallel, 1 perpendicular
extrude "Extrusion16" cut sketch "Sketch15" against normal blind 4
sketch "Sketch16" plane through (29.095, 1.6, 10.275) normal (1, 0, 0) x (0, 0, -1)
  line L0 (28.05, -4.1) -> (-7.5, -4.1) projected
  line L1 (-7.5, 0) -> (28.05, 0)
  line L2 (28.05, 0) -> (28.05, -4.1)
  line L3 (28.05, -4.1) -> (-7.5, -4.1)
  line L4 (-7.5, -4.1) -> (-7.5, 0)
  point P0 (10.275, -1.6)
  constraints: 8 end point, 2 parallel, 1 horizontal, 1 perpendicular
extrude "Extrusion17" add sketch "Sketch16" along normal blind 5
sketch "Sketch17" plane through (-21.595, 1.6, 17.775) normal (0, 0, 1) x (1, 0, 0)
  line L0 (-7.5, -4.1) -> (-7.5, 0) projected
  line L1 (-7.5, -4.1) -> (55.69, -4.1) projected
  line L2 (-7.5, 0) -> (55.69, 0)
  line L3 (55.69, 0) -> (55.69, -4.1)
  line L4 (55.69, -4.1) -> (-7.5, -4.1)
  line L5 (-7.5, -4.1) -> (-7.5, 0)
  point P0 (21.595, -1.6)
  constraints: 8 end point, 2 parallel, 1 horizontal, 1 perpendicular
extrude "Extrusion18" add sketch "Sketch17" along normal blind 5
sketch "Sketch18" plane through (21.595, 1.6, -17.775) normal (0, 0, -1) x (-1, 0, 0)
  line L0 (50.69, 0) -> (-12.5, 0) projected
  line L1 (50.69, -4.1) -> (-12.5, -4.1) projected
  line L2 (-12.5, 0) -> (50.69, 0)
  line L3 (50.69, 0) -> (50.69, -4.1)
  line L4 (50.69, -4.1) -> (-12.5, -4.1)
  line L5 (-12.5, -4.1) -> (-12.5, 0)
  point P0 (21.595, -1.6)
  constraints: 8 end point, 2 parallel, 1 horizontal, 1 perpendicular
extrude "Extrusion19" add sketch "Sketch18" along normal blind 5
sketch "Sketch19" plane through (0, 1.6, 0) normal (0, 1, 0) x (1, 0, 0)
  line L0 (-26.595, 20.275) -> (-24.095, 20.275)
  line L1 (-24.095, 17.775) -> (-26.595, 17.775)
  line L2 (-26.5, 20.275) -> (26.5, 20.275)
  line L3 (26.5, 17.775) -> (-26.5, 17.775)
  line L4 (-26.5, 17.775) -> (-26.5, 20.275)
  line L5 (-26.5, 20.275) -> (26.5, 17.775) construction
  line L6 (26.5, 20.275) -> (-26.5, 17.775) construction
  line L7 (26.5, 17.775) -> (30.5, 17.775)
  line L8 (30.5, 17.775) -> (30.5, 20.275)
  line L9 (30.5, 20.275) -> (26.5, 20.275)
  line L10 (-26.5, 20.275) -> (30.5, 20.275)
  line L11 (30.5, 20.275) -> (30.5, 17.775)
  line L12 (30.5, 17.775) -> (-26.5, 17.775)
  line L13 (-26.5, 17.775) -> (-26.5, 20.275)
  line L14 (-25.095, 13.775) -> (25.095, 13.775) projected
  line L15 (0, 13.775) -> (0, 0)
  line L16 (0, 0) -> (0, -13.775)
  line L17 (25.095, -13.775) -> (-25.095, -13.775) projected
  line L18 (0, 13.775) -> (0, 19.025)
  line L19 (0, -13.775) -> (0, -19.025)
  line L20 (26.5, -17.775) -> (-26.5, -17.775)
  line L21 (-26.5, -17.775) -> (-26.5, -20.275)
  line L22 (-26.5, -20.275) -> (26.5, -20.275)
  line L23 (26.5, -17.775) -> (-26.5, -20.275) construction
  line L24 (-26.5, -17.775) -> (26.5, -20.275) construction
  line L25 (26.5, -20.275) -> (30.5, -20.275)
  line L26 (30.5, -20.275) -> (30.5, -17.775)
  line L27 (30.5, -17.775) -> (26.5, -17.775)
  line L28 (-26.5, -20.275) -> (30.5, -20.275)
  line L29 (30.5, -20.275) -> (30.5, -17.775)
  line L30 (30.5, -17.775) -> (-26.5, -17.775)
  line L31 (-26.5, -17.775) -> (-26.5, -20.275)
  dimension "d181" = 53
  dimension "d182" = 2.5
  dimension "d183" = 4
  dimension "d185" = 5.25
  dimension "d186" = 2.5
  constraints: 60 end point, 9 parallel, 7 horizontal, 6 midpoint, 6 perpendicular, 1 point on line, 1 vertical
  measures "d181" distance of L3.start L3.end
  measures "d182" distance between parallel lines of L2 L3
  measures "d183" distance of L9.end L8.end
  measures "d185" distance of L16.end L19.end
  measures "d186" distance of L21.end L20.end
extrude "Extrusion20" add sketch "Sketch19" along normal blind 3
sketch "Sketch20" plane through (34.095, 1.6, 10.275) normal (1, 0, 0) x (0, 0, -1)
  line L0 (33.05, 0) -> (-12.5, 0) projected
  line L1 (18.55, -4.1) -> (33.05, -4.1) projected
  line L2 (-12.5, 0) -> (33.05, 0)
  line L3 (33.05, 0) -> (33.05, -4.1)
  line L4 (33.05, -4.1) -> (-12.5, -4.1)
  line L5 (-12.5, -4.1) -> (-12.5, 0)
  point P0 (10.275, -1.6)
  constraints: 8 end point, 2 parallel, 1 horizontal, 1 perpendicular
extrude "Extrusion21" add sketch "Sketch20" along normal blind 10
sketch "Sketch21" plane through (0, -2.5, 0) normal (0, -1, 0) x (1, 0, 0)
  line L0 (-29.095, -22.775) -> (44.095, -22.775) projected
  line L1 (44.095, -22.775) -> (-29.095, -22.775)
  line L2 (-29.095, -22.775) -> (-29.095, 22.775)
  line L3 (-29.095, 22.775) -> (44.095, 22.775)
  line L4 (44.095, 22.775) -> (44.095, -22.775)
  line L5 (-16.095, -8.275) -> (-29.095, -8.275) projected
  line L6 (-29.095, 8.275) -> (-16.095, 8.275) projected
  line L7 (-16.095, -8.275) -> (-29.095, -8.275)
  line L8 (-29.095, -8.275) -> (-29.095, 8.275)
  line L9 (-29.095, 8.275) -> (-16.095, 8.275)
  line L10 (-16.095, 8.275) -> (-16.095, -8.275)
  line L11 (-23.3003, 11.9803) -> (-19.8897, 11.9803)
  line L12 (-19.8897, 11.9803) -> (-19.8897, 8.275)
  line L13 (-19.8897, 8.275) -> (-23.3003, 8.275)
  line L14 (-23.3003, 8.275) -> (-23.3003, 11.9803)
  line L15 (-23.3003, 11.9803) -> (-24.3003, 11.9803)
  line L16 (-24.3003, 11.9803) -> (-24.3003, 8.275)
  line L17 (-24.3003, 8.275) -> (-23.3003, 8.275)
  line L18 (-23.3003, 8.275) -> (-23.3003, 11.9803)
  line L19 (-19.8897, 11.9803) -> (-18.8897, 11.9803)
  line L20 (-18.8897, 11.9803) -> (-18.8897, 8.275)
  line L21 (-18.8897, 8.275) -> (-19.8897, 8.275)
  line L22 (-19.8897, 8.275) -> (-19.8897, 11.9803)
  line L23 (-24.3003, 11.9803) -> (-18.8897, 11.9803)
  line L24 (-18.8897, 11.9803) -> (-18.8897, 12.9803)
  line L25 (-18.8897, 12.9803) -> (-24.3003, 12.9803)
  line L26 (-24.3003, 12.9803) -> (-24.3003, 11.9803)
  line L27 (-19.8897, -11.9803) -> (-23.3003, -11.9803)
  line L28 (-23.3003, -11.9803) -> (-23.3003, -8.275)
  line L29 (-23.3003, -8.275) -> (-19.8897, -8.275)
  line L30 (-19.8897, -8.275) -> (-19.8897, -11.9803)
  line L31 (-23.3003, -8.275) -> (-24.3003, -8.275)
  line L32 (-24.3003, -8.275) -> (-24.3003, -11.9803)
  line L33 (-24.3003, -11.9803) -> (-23.3003, -11.9803)
  line L34 (-23.3003, -11.9803) -> (-23.3003, -8.275)
  line L35 (-19.8897, -11.9803) -> (-18.8897, -11.9803)
  line L36 (-18.8897, -11.9803) -> (-18.8897, -8.275)
  line L37 (-18.8897, -8.275) -> (-19.8897, -8.275)
  line L38 (-19.8897, -8.275) -> (-19.8897, -11.9803)
  line L39 (-18.8897, -11.9803) -> (-24.3003, -11.9803)
  line L40 (-24.3003, -11.9803) -> (-24.3003, -12.9803)
  line L41 (-24.3003, -12.9803) -> (-18.8897, -12.9803)
  line L42 (-18.8897, -12.9803) -> (-18.8897, -11.9803)
  point P0 (0, 0)
  dimension "d143" = 1
  dimension "d144" = 1
  dimension "d145" = 1
  dimension "d146" = 1
  constraints: 80 end point, 20 parallel, 12 point on line, 10 horizontal, 10 perpendicular
  measures "d143" distance of L17.end L16.end
  measures "d144" distance of L20.end L21.end
  measures "d145" distance of L24.end L23.end
  measures "d146" distance of L40.end L39.end
extrude "Extrusion22" add sketch "Sketch21" along normal blind 2 contours L2 L5 L32 L40 L41 L42 L36 L10 L6 L20 L24 L25 L26 L16 L3 L4 L0
fillet "Fillet3" radius 5 4 edges at (44.095, -1.45, -22.775) (44.095, -1.45, 22.775) (-29.095, -1.45, 22.775) (-29.095, -1.45, -22.775)
fillet "Fillet4" radius 2 9 edges at (44.095, -4.5, 0) (42.6305, -4.5, 21.3105) (7.5, -4.5, 22.775) (-27.6305, -4.5, 21.3105) (-29.095, -4.5, 13.025) (42.6305, -4.5, -21.3105) (7.5, -4.5, -22.775) (-27.6305, -4.5, -21.3105) (-29.095, -4.5, -13.025)
sketch "Sketch24" plane through (0, -2.4, 0) normal (0, 1, 0) x (1, 0, 0)
  line L0 (-16.095, -8.275) -> (-16.095, 8.275) projected
  line L1 (-16.095, 8.275) -> (21.905, 8.275)
  line L2 (21.905, 8.275) -> (21.905, -8.275)
  line L3 (21.905, -8.275) -> (-16.095, -8.275)
  line L4 (-16.095, -8.275) -> (-16.095, 8.275)
  point P0 (0, 0)
  dimension "d157" = 38
  constraints: 8 end point, 2 parallel, 1 horizontal, 1 perpendicular
  measures "d157" distance of L2.end L3.end
extrude "Extrusion24" cut sketch "Sketch24" against normal blind 2.5
fillet "Fillet5" radius 2 4 edges at (25.095, -0.4, -13.775) (25.095, -0.4, 13.775) (-25.095, -0.4, 13.775) (-25.095, -0.4, -13.775)
sketch "Sketch26" plane through (0, -2.5, 0) normal (0, -1, 0) x (1, 0, 0)
  line L0 (-24.3003, 12.9803) -> (-24.3003, 8.275) projected
  line L1 (-18.8897, 8.275) -> (-18.8897, 12.9803) projected
  line L2 (-24.3003, 12.9803) -> (-18.8897, 12.9803)
  line L3 (-18.8897, 12.9803) -> (-18.8897, 8.275)
  line L4 (-18.8897, 8.275) -> (-24.3003, 8.275)
  line L5 (-24.3003, 8.275) -> (-24.3003, 12.9803)
  line L6 (-18.8897, -12.9803) -> (-18.8897, -8.275) projected
  line L7 (-18.8897, -8.275) -> (-24.3003, -8.275)
  line L8 (-24.3003, -8.275) -> (-24.3003, -12.9803)
  line L9 (-24.3003, -12.9803) -> (-18.8897, -12.9803)
  line L10 (-18.8897, -12.9803) -> (-18.8897, -8.275)
  point P0 (0, 0)
  constraints: 16 end point, 4 parallel, 2 horizontal, 2 perpendicular, 1 point on line
extrude "Extrusion26" add sketch "Sketch26" along normal blind 2
sketch "Sketch27" plane through (-21.595, -2.5, -10.275) normal (0, 1, 0) x (1, 0, 0)
  circle A0 centre (0, 0) radius 1
  circle A1 centre (0, -20.55) radius 1.7053 projected
  circle A2 centre (0, -20.55) radius 1
  point P0 (21.595, -10.275)
  dimension "d166" = 2
  dimension "d167" = 2
  constraints: 2 centre point, 1 coincident
  measures "d166" diameter of A0
  measures "d167" diameter of A2
extrude "Extrusion27" add sketch "Sketch27" along normal blind 4 contours A0 | A2
fillet "Fillet6" radius 1 2 edges at (-22.595, 1.5, 10.275) (-22.595, 1.5, -10.275)
sketch "Sketch28" plane through (21.905, -2.4, -8.275) normal (-1, 0, 0) x (0, 0, 1)
  line L0 (16.55, -2.1) -> (0, -2.1) projected
  line L1 (16.55, -2.1) -> (16.55, -0.1) projected
  line L2 (0, -2.1) -> (16.55, -2.1)
  line L3 (16.55, -2.1) -> (16.55, -0.1)
  line L4 (16.55, -0.1) -> (0, -0.1)
  line L5 (0, -0.1) -> (0, -2.1)
  point P0 (8.275, 2.4)
  constraints: 8 end point, 2 parallel, 1 horizontal, 1 perpendicular
extrude "Extrusion28" add sketch "Sketch28" along normal blind 40
sketch "Sketch29" plane through (21.905, -2.5, 8.275) normal (0, 1, 0) x (1, 0, 0)
  line L0 (0, 16.55) -> (0, 0) projected
  line L1 (-40, 16.55) -> (-40, 0) projected
  line L2 (0, 16.55) -> (-40, 16.55)
  line L3 (-40, 16.55) -> (-40, 0)
  line L4 (-40, 0) -> (0, 0)
  line L5 (0, 0) -> (0, 16.55)
  point P0 (-21.905, 8.275)
  constraints: 8 end point, 2 parallel, 1 horizontal, 1 perpendicular
extrude "Extrusion29" cut sketch "Sketch29" along normal blind 1
sketch "Sketch30" plane through (21.905, -2.5, 8.275) normal (0, 1, 0) x (1, 0, 0)
  line L0 (0, 0) -> (-40, 0) projected
  line L1 (-40, 16.55) -> (-40, 0) projected
  line L2 (0, 0) -> (-40, 0)
  line L3 (-40, 0) -> (-40, 16.55)
  line L4 (-40, 16.55) -> (0, 16.55)
  line L5 (0, 16.55) -> (0, 0)
  point P0 (-21.905, 8.275)
  constraints: 8 end point, 2 parallel, 1 horizontal, 1 perpendicular
extrude "Extrusion30" cut sketch "Sketch30" against normal blind 1
sketch "Sketch31" plane through (-29.095, -0.4, -8.275) normal (0, -1, 0) x (1, 0, 0)
  line L0 (0, 0) -> (2, 0) projected
  line L1 (0, 16.55) -> (4, 16.55) projected
  line L2 (0, 0) -> (4, 0)
  line L3 (4, 0) -> (4, 16.55)
  line L4 (4, 16.55) -> (0, 16.55)
  line L5 (0, 16.55) -> (0, 0)
  point P0 (29.095, 8.275)
  constraints: 8 end point, 2 parallel, 1 horizontal, 1 perpendicular
extrude "Extrusion31" cut sketch "Sketch31" against normal blind 2